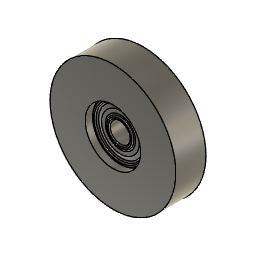
F0850-12 v1 (Autodesk Fusion 360 design; units mm, degrees)
Autodesk Fusion 360 part; units mm, degrees
note: some values were not read from the file. Set by a fixed rule: which sketch regions a step uses.
sketch "Sketch1" plane through (0, 0, 0) normal (1, 0, 0) x (0, 1, 0)
  line L0 (-6, 0) -> (6, 0)
  line L1 (6, 0) -> (6, 14)
  line L2 (6, 14) -> (-6, 14)
  line L3 (-6, 14) -> (-6, 0)
  line L4 (-3.5, 21) -> (3.5, 21) construction
  line L5 (3.5, 21) -> (3.5, 14) construction
  line L6 (3.5, 14) -> (-3.5, 14) construction
  line L7 (-3.5, 14) -> (-3.5, 21) construction
  line L8 (0, 21) -> (0, 29) construction
  line L9 (3.5, 19.6) -> (-3.5, 19.6)
  line L10 (3.5, 15.4) -> (-3.5, 15.4) construction
  circle A0 centre (0, 17.5) radius 2.5
  line L11 (3.5, 15.4) -> (3.075, 15.4) construction
  line L12 (3.075, 15.4) -> (3.075, 14.975) construction
  circle A1 centre (3.075, 14.975) radius 0.425
  line L13 (3.075, 15.4) -> (3.075, 15.1875)
  line L14 (3.075, 15.1875) -> (2.6876, 14.8001)
  line L15 (2.6876, 14.8001) -> (2.0878, 15.4)
  line L16 (2.0878, 15.4) -> (1.3565, 15.4)
  line L17 (-3.5, 15.4) -> (-3.075, 15.4) construction
  line L18 (-3.075, 15.4) -> (-3.075, 14.975) construction
  circle A2 centre (-3.075, 14.975) radius 0.425
  line L19 (-3.075, 15.4) -> (-3.075, 15.1875)
  line L20 (-3.075, 15.1875) -> (-2.6876, 14.8001)
  line L21 (-3.075, 15.1875) -> (-2.5272, 15.1875) construction
  line L22 (-2.6876, 14.8001) -> (-2.0878, 15.4)
  line L23 (-2.0878, 15.4) -> (-1.3565, 15.4)
  line L24 (-3.5, 25) -> (3.5, 25) construction
  line L25 (-3.5, 19.6) -> (-3.075, 19.6) construction
  line L26 (-3.075, 19.6) -> (-3.075, 20.025) construction
  circle A3 centre (-3.075, 20.025) radius 0.425
  line L27 (3.5, 14) -> (3.075, 14) construction
  line L28 (3.075, 14) -> (3.075, 14.425) construction
  circle A4 centre (3.075, 14.425) radius 0.425
  line L29 (-3.5, 14) -> (-3.075, 14) construction
  line L30 (-3.075, 14) -> (-3.075, 14.425) construction
  circle A5 centre (-3.075, 14.425) radius 0.425
  line L31 (-3.5, 21) -> (-3.075, 21) construction
  line L32 (-3.075, 21) -> (-3.075, 20.575) construction
  circle A6 centre (-3.075, 20.575) radius 0.425
  line L33 (3.5, 15.4) -> (3.5, 14)
  line L34 (-3.5, 15.4) -> (-3.5, 14)
  line L35 (-3.5, 19.6) -> (-3.5, 21) construction
  line L36 (3.5, 21) -> (3.075, 21) construction
  line L37 (3.075, 21) -> (3.075, 20.575) construction
  line L38 (3.5, 19.6) -> (3.075, 19.6) construction
  line L39 (3.075, 19.6) -> (3.075, 20.025) construction
  line L40 (3.5, 19.6) -> (3.5, 21)
  circle A7 centre (3.075, 20.025) radius 0.425
  circle A8 centre (3.075, 20.575) radius 0.425
  line L41 (-3.5, 21) -> (3.5, 21)
  line L42 (3.075, 15.4) -> (2.7, 16)
  line L43 (2.7, 16) -> (2.9989, 17.5)
  line L44 (2.9989, 17.5) -> (2.9989, 19)
  line L45 (2.9989, 19) -> (3.075, 19.6)
  line L46 (-3.075, 15.4) -> (-2.7, 16)
  line L47 (-2.7, 16) -> (-3, 17.5)
  line L48 (-3, 17.5) -> (-3, 19)
  line L49 (-3, 19) -> (-3.075, 19.6)
  line L50 (-3.5, 19.6) -> (-3.5, 21)
  dimension "d2" = 12
  dimension "d3" = 14
  dimension "d4" = 7
  dimension "d5" = 7
  dimension "d6" = 8
  dimension "d11" = 1.4
  dimension "d12" = 1.4
  dimension "d13" = 5
  dimension "d14" = 0.425
  dimension "d15" = 0.425
  dimension "d16" = 135
  dimension "d17" = 0.425
  dimension "d18" = 0.425
  dimension "d19" = 45
  dimension "d20" = 0.425
  dimension "d21" = 0.425
  dimension "d22" = 0.425
  dimension "d23" = 0.425
  dimension "d24" = 0.425
  dimension "d25" = 0.425
  dimension "d26" = 0.425
  dimension "d27" = 0.425
  dimension "d28" = 0.425
  dimension "d29" = 0.425
  dimension "d30" = 0.425
  dimension "d31" = 0.425
  constraint horizontal L0
  constraint vertical L1
  constraint horizontal L2
  constraint vertical L3
  constraint horizontal L4
  constraint vertical L5
  constraint horizontal L6
  constraint vertical L7
  constraint midpoint L4 L8.start
  constraint perpendicular L4 L8
  constraint coincident L7 L9.end
  constraint perpendicular L7 L9
  constraint perpendicular L5 L11
  constraint perpendicular L10 L12
  constraint coincident L12.end A1.centre
  constraint coincident L11.end A1
  constraint tangent L10 A1
  constraint midpoint L12 L13.end
  constraint coincident A1 L14.end
  constraint coincident L10 L15.end
  constraint perpendicular L14 L15
  constraint coincident A0 L16.end
  constraint coincident L10 L16.end
  constraint perpendicular L7 L17
  constraint perpendicular L10 L18
  constraint coincident L18.end A2.centre
  constraint coincident L17.end A2
  constraint midpoint L18 L19.end
  constraint horizontal L21
  constraint coincident A2 L20.end
  constraint coincident L10 L22.end
  constraint perpendicular L20 L22
  constraint coincident L10 L23.end
  constraint coincident A0 L23.end
  constraint horizontal L24
  constraint midpoint L8 L24
  constraint coincident L9 L25.end
  constraint perpendicular L25 L26
  constraint coincident L26.end A3.centre
  constraint coincident L25.end A3
  constraint perpendicular L5 L27
  constraint perpendicular L2 L28
  constraint coincident L28.end A4.centre
  constraint coincident L27.end A4
  constraint perpendicular L6 L30
  constraint coincident L30.end A5.centre
  constraint coincident L29.end A5
  constraint perpendicular L7 L31
  constraint perpendicular L31 L32
  constraint coincident L32.end A6.centre
  constraint coincident L31.end A6
  constraint perpendicular L10 L33
  constraint perpendicular L6 L34
  constraint perpendicular L5 L36
  constraint perpendicular L4 L37
  constraint perpendicular L5 L38
  constraint perpendicular L38 L39
  constraint perpendicular L4 L40
  constraint coincident L39.end A7.centre
  constraint coincident L38.end A7
  constraint coincident L37.end A8.centre
  constraint coincident L36.end A8
  constraint perpendicular L11 L44
  constraint vertical L48
  measures "d2" distance of L0.start L0.end
  measures "d3" distance of L0.start L2.end
  measures "d4" distance of L4.start L4.end
  measures "d5" distance of L4.start L6.end
  measures "d6" distance of L8.start L8.end
  measures "d11" distance of L4.end L9.start
  measures "d12" distance of L5.end L10.start
  measures "d13" diameter of A0
  measures "d14" distance of L10.start L11.end
  measures "d15" distance of L11.end L12.end
  measures "d16" angle of L13 L14
  measures "d17" distance of L10.end L17.end
  measures "d18" distance of L17.end L18.end
  measures "d19" angle of L20 L21
  measures "d20" distance of L9.end L25.end
  measures "d21" distance of L25.end L26.end
  measures "d22" distance of L5.end L27.end
  measures "d23" distance of L27.end L28.end
  measures "d24" distance of L6.end L29.end
  measures "d25" distance of L29.end L30.end
  measures "d26" distance of L4.start L31.end
  measures "d27" distance of L31.end L32.end
  measures "d28" distance of L4.end L36.end
  measures "d29" distance of L36.end L37.end
  measures "d30" distance of L9.start L38.end
  measures "d31" distance of L38.end L39.end
revolve "Revolve1" add sketch "Sketch1" angle 360 about axis through (0, -3.5, 25) along (0, 1, 0) contours L2 A0 A1 L15 L16 A2 L22 L23 A4 A5 | A2 A5 | A2 A5 L34 | A1 A4 | A1 A4 L33 | A2 A5 | A2 L19 L20 A5 | A1 A4 | A1 L13 L14 A4 | L9 A0 A2 L22 L23 L46 L47 L48 L49 | A2 L19 L20 | L9 A0 A1 L15 L16 L42 L43 L44 L45 | A1 L13 L14 | L9 A0 A3 A6 A7 A8 L41 | A3 A6 | A7 A8 | A3 A6 L50 | L40 A7 A8 | A7 A8 | A7 A8 | A3 A6 | A3 A6
revolve "Revolve2" add sketch "Sketch1" angle 360 about axis through (0, -3.5, 25) along (0, 1, 0) contours L0 L1 L2 L3
